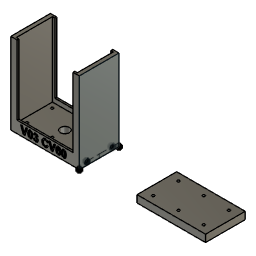
KaiserStandBracket 4 CV60 v5 (Autodesk Fusion 360 design; units mm, degrees)
Autodesk Fusion 360 part; units mm, degrees
sketch "Schizzo1" plane through (0, 0, 0) normal (0, 0, 1) x (1, 0, 0)
  line L0 (164.882, 47.8317) -> (240.882, 47.8317)
  line L1 (240.882, 47.8317) -> (240.882, 3.8317)
  line L2 (240.882, 3.8317) -> (164.882, 3.8317)
  line L3 (164.882, 3.8317) -> (164.882, 47.8317)
  line L4 (202.882, 47.8317) -> (202.882, 3.8317) construction
  circle A0 centre (202.882, 39.8317) radius 1.4
  line L5 (164.882, 25.8317) -> (240.882, 25.8317) construction
  circle A1 centre (202.882, 11.8317) radius 1.4
  circle A2 centre (174.882, 11.8317) radius 1.4
  circle A3 centre (174.882, 39.8317) radius 1.4
  circle A4 centre (230.882, 11.8317) radius 1.4
  circle A5 centre (230.882, 39.8317) radius 1.4
  circle A6 centre (202.882, 25.8317) radius 5
  line L6 (164.882, 45.8317) -> (240.882, 45.8317)
  line L7 (164.882, 5.8317) -> (240.882, 5.8317)
  line L8 (169.082, 45.8317) -> (169.082, 5.8317)
  line L9 (236.682, 45.8317) -> (236.682, 5.8317)
  line L10 (171.882, 47.8317) -> (171.882, 45.8317)
  line L11 (233.882, 47.8317) -> (233.882, 45.8317)
  line L12 (171.882, 3.8317) -> (171.882, 5.8317)
  line L13 (233.882, 3.8317) -> (233.882, 5.8317)
  circle A7 centre (342.882, 39.8317) radius 1.4
  line L14 (304.882, 3.8317) -> (304.882, 47.8317)
  circle A8 centre (314.882, 11.8317) radius 1.4
  circle A9 centre (342.882, 11.8317) radius 1.4
  line L15 (342.882, 47.8317) -> (342.882, 3.8317) construction
  circle A10 centre (370.882, 39.8317) radius 1.4
  line L16 (304.882, 25.8317) -> (380.882, 25.8317) construction
  line L17 (380.882, 3.8317) -> (304.882, 3.8317)
  circle A11 centre (370.882, 11.8317) radius 1.4
  line L18 (380.882, 47.8317) -> (380.882, 3.8317)
  circle A12 centre (314.882, 39.8317) radius 1.4
  line L19 (304.882, 47.8317) -> (380.882, 47.8317)
  dimension "d44" = 76
  dimension "d45" = 44
  dimension "d46" = 2.8
  dimension "d47" = 28
  dimension "d50" = 28
  dimension "d51" = 0
  dimension "d54" = 10
  dimension "d55" = 2
  dimension "d56" = 4.2
  dimension "d57" = 7
  dimension "d76" = 28
  dimension "d77" = 0
  dimension "d78" = 76
  dimension "d79" = 44
  dimension "d80" = 2.8
  dimension "d81" = 28
  constraint horizontal L0
  constraint vertical L1
  constraint horizontal L2
  constraint vertical L3
  constraint midpoint L0 L4.start
  constraint midpoint L2 L4.end
  constraint coincident L4 A0.centre
  constraint midpoint L3 L5.start
  constraint midpoint L1 L5.end
  constraint symmetric A0 L5 A1
  constraint midpoint L4 A6.centre
  constraint coincident L3 L6.start
  constraint coincident L1 L6.end
  constraint perpendicular L1 L6
  constraint symmetric L5 L6.start L7.start
  constraint symmetric L5 L6.end L7.end
  constraint coincident L6 L8.start
  constraint coincident L7 L8.end
  constraint perpendicular L7 L8
  constraint symmetric L4 L8.start L9.start
  constraint symmetric L4 L8.end L9.end
  constraint coincident L0 L10.start
  constraint coincident L6 L10.end
  constraint perpendicular L6 L10
  constraint symmetric L4 L10.start L11.start
  constraint symmetric L4 L10.end L11.end
  constraint symmetric L5 L10.start L12.start
  constraint symmetric L5 L10.end L12.end
  constraint symmetric L5 L11.start L13.start
  constraint symmetric L5 L11.end L13.end
  constraint horizontal L19
  constraint vertical L18
  constraint horizontal L17
  constraint vertical L14
  constraint midpoint L15.start L19
  constraint midpoint L15.end L17
  constraint coincident A7.centre L15
  constraint midpoint L16.start L14
  constraint midpoint L16.end L18
  constraint symmetric A7 A9 L16
  measures "d44" distance of L0.start L0.end
  measures "d45" distance of L0.start L2.end
  measures "d46" diameter of A0
  measures "d47" distance of A0.centre A1.centre
  measures "d54" diameter of A6
  measures "d55" distance of L0 L6
  measures "d56" distance of L3 L8
  measures "d57" distance of L3 L10
  measures "d78" distance of L14.end L18.start
  measures "d79" distance of L14.end L14.start
  measures "d80" diameter of A7
  measures "d81" distance of A7.centre A9.centre
extrude "Estrusione8" add sketch "Schizzo1" along normal blind 8 contours L0 L3 L6 L10 | L0 L6 L10 L11 | L3 L6 L7 L8 | L0 L1 L6 L11 | L6 L7 L8 L9 | L2 L3 L7 L12 | L1 L6 L7 L9 | L2 L7 L12 L13 | L1 L2 L7 L13 makes body 1
extrude "Estrusione9" add sketch "Schizzo1" along normal blind 90 contours L0 L3 L6 L10 | L3 L6 L7 L8 | L0 L1 L6 L11 | L2 L3 L7 L12 | L1 L6 L7 L9 | L1 L2 L7 L13 bodies 1
extrude "Estrusione10" add sketch "Schizzo1" along normal blind 5 from surface at 8 contours L0 L6 L10 L11 | L2 L7 L12 L13 bodies 1
sketch "Schizzo4" plane through (0, 3.8317, 0) normal (0, -1, 0) x (1, 0, 0)
  line L0 (171.882, 13) -> (171.882, 90)
  line L1 (171.882, 90) -> (164.882, 90)
  line L2 (164.882, 90) -> (164.882, 0)
  line L3 (164.882, 0) -> (240.882, 0)
  line L4 (240.882, 0) -> (240.882, 90)
  line L5 (240.882, 90) -> (233.882, 90)
  line L6 (233.882, 90) -> (233.882, 13)
  line L7 (233.882, 13) -> (171.882, 13)
  line L8 (175.9241, 2.0872) -> (235.2612, 2.0872) construction
  line L9 (235.2612, 2.0872) -> (235.2612, 10.7343) construction
  line L10 (235.2612, 10.7343) -> (175.9241, 10.7343) construction
  line L11 (175.9241, 10.7343) -> (175.9241, 2.0872) construction
  dimension "d63" = 8
  text T0 "V03 CV60" font "Arial" height 8 bold align left top in box 59.3371 x 8.6471 at (175.9241, 2.0872) x (1, 0) y (0, 1) spacing 1
extrude "Estrusione11" cut sketch "Schizzo4" against normal blind 1 text T0 bodies 1
sketch "Schizzo5" plane through (240.882, 0, 0) normal (1, 0, 0) x (0, 1, 0)
  line L0 (3.8317, 0) -> (47.8317, 0)
  line L1 (47.8317, 0) -> (47.8317, 90)
  line L2 (47.8317, 90) -> (3.8317, 90)
  line L3 (3.8317, 90) -> (3.8317, 0)
  line L4 (3.8317, 0) -> (47.8317, 0) construction
  line L5 (47.8317, 0) -> (47.8317, 4) construction
  line L6 (47.8317, 4) -> (3.8317, 4) construction
  line L7 (3.8317, 4) -> (3.8317, 0) construction
  line L8 (25.8317, 4) -> (25.8317, 0) construction
  circle A0 centre (11.8317, 4) radius 1.4
  circle A1 centre (39.8317, 4) radius 1.4
  dimension "d66" = 4
  dimension "d67" = 2.8
  dimension "d68" = 28
  constraint horizontal L4
  constraint vertical L5
  constraint horizontal L6
  constraint vertical L7
  constraint coincident L0.start L3.end
  constraint coincident L0.end L1.start
  constraint midpoint L6 L8.start
  constraint midpoint L4 L8.end
  constraint coincident L6 A0.centre
  constraint symmetric L8 A0 A1
  measures "d66" distance of L4 L6
  measures "d67" diameter of A0
  measures "d68" distance of A0.centre A1.centre
extrude "Estrusione12" cut sketch "Schizzo5" against normal blind 10 contours A0 | A1 bodies 1
extrude "Estrusione13" cut sketch "Schizzo5" along normal blind 10 from surface at -76 contours A0 | A1 bodies 1
extrude "Estrusione14" add sketch "Schizzo1" along normal blind 8 separate body contours L14 L17 L18 L19 makes body 2
